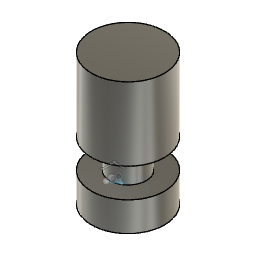
Valitin v3 (Autodesk Fusion 360 design; units mm, degrees)
Autodesk Fusion 360 part; units mm, degrees
cylinder "CylinderPrimitive1" add diameter 5 height 2 placed x (1, 0, 0) y (0, 1, 0) z (0, 0, 1) at (0, 0, 0)
cylinder "CylinderPrimitive2" add diameter 2.5 height 2 placed x (1, 0, 0) y (0, 1, 0) z (0, 0, 1) at (0, 0, 2)
cylinder "CylinderPrimitive3" add diameter 5 height 5 placed x (1, 0, 0) y (0, 1, 0) z (0, 0, 1) at (0, 0, 4)
hole "Hole1" at (0, 0, 0) direction (0, 0, 1) diameter 2 depth 1 tip angle 180
sketch "Sketch5" plane through (0, 0, 1) normal (0, 0, -1) x (1, 0, 0)
  circle A0 centre (0, 0) radius 1
  line L0 (-1, 0.0018) -> (-0.4102, 0.0018)
  line L1 (-0.4102, 0.0018) -> (-1.1, 0.4)
  line L2 (-0.4102, 0.0018) -> (-0.9506, -0.3103)
  line L3 (-0.4102, 0.0018) -> (-1.1146, 0.0018) construction
  dimension "d10" = 30
  dimension "d11" = 30
  constraint coincident A0 L0.start
  constraint horizontal L0
  constraint horizontal L3
  constraint coincident A0 L2.end
  measures "d10" angle of L0 L1
  measures "d11" angle of L2 L3
extrude "Extrude1" add sketch "Sketch5" along normal blind 1 contours A0 L0 L1
extrude "Extrude2" add sketch "Sketch5" along normal blind 1 contours A0 L0 L2
pattern_circular "C-Pattern1" count 10 over 360 about axis through (0, 0, 2) along (0, 0, 1) of 2 faces at (-0.59, -0.1056, 0.6667) (-0.5904, 0.1023, 0.6667)
